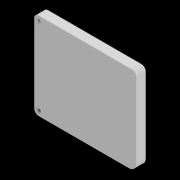
# Autodesk Inventor part: switchback-logo-cover
Saved by Autodesk Inventor 2020 (Build 240168000, 168)
## iProperties
Created: 2020-02-04
Part Number: switchback-logo-cover
Material: Generic
Document SubType Name: Modeling
Designer: valer
Density: 1 g/cm^3
Appearance: Default
Author: valer
Autodesk Inventor part; units mm, degrees
ref_plane "YZ Plane" through (0, 0, 0) normal (1, 0, 0) x (0, 1, 0)
ref_plane "XZ Plane" through (0, 0, 0) normal (0, 1, 0) x (-1, 0, 0)
ref_plane "XY Plane" through (0, 0, 0) normal (0, 0, 1) x (1, 0, 0)
sketch "Base" plane through (0, 0, 0) normal (0, 0, 1) x (1, 0, 0)
  circle A0 centre (1.3558, 26.9285) radius 0.635
  line L0 (1.5304, 28.5212) -> (33.5414, 28.5212)
  spline S0 degree 3 poles (-0.2127, 27.3007) (-0.2118, 27.3054) (-0.211, 27.3101) (-0.1754, 27.4946) (-0.1031, 27.6795) (0.1087, 28.0058) (0.2483, 28.1472) (0.5483, 28.3572) (0.7287, 28.4399) (1.0276, 28.5086) (1.1402, 28.5212) (1.2508, 28.5212) knots 0.443162 0.443162 0.443162 0.443162 0.444594 0.444594 0.49954 0.49954 0.554486 0.554486 0.609433 0.609433 0.641273 0.641273 0.641273 0.641273
  ellipse E0 centre (1.2507, 27.0333) end of major axis (1.2953, 25.5461) minor radius 1.4876 (-0.2127, 27.3007) -> (-0.2369, 27.0333) ccw
  line L1 (-0.2366, -0.0071) -> (-0.2369, 27.0333)
  ellipse E1 centre (33.5414, 27.0636) end of major axis (33.5851, 25.6066) minor radius 1.4573 (34.9987, 27.0636) -> (33.5414, 28.5212) ccw
  line L2 (34.9987, 27.0636) -> (34.999, 1.0356)
  circle A1 centre (33.7947, 27.0657) radius 0.635
  ellipse E2 centre (32.4689, 1.0356) end of major axis (32.5448, -1.4939) minor radius 2.5301 (32.469, -1.495) -> (34.999, 1.0356) ccw
  line L3 (32.469, -1.495) -> (1.251, -1.495)
  ellipse E3 centre (1.251, -0.0071) end of major axis (1.2956, -1.4943) minor radius 1.4876 (-0.2366, -0.0071) -> (1.251, -1.495) ccw
  circle A2 centre (1.3611, 0.1027) radius 0.635
  line L4 (1.2508, 28.5212) -> (1.5304, 28.5212)
  point P0 (0, 0)
  constraints: 10 end point, 3 centre point, 1 horizontal, 18 other
extrude "BaseFeature" add sketch "Base" along normal blind 3.2004
body "Solid1"
